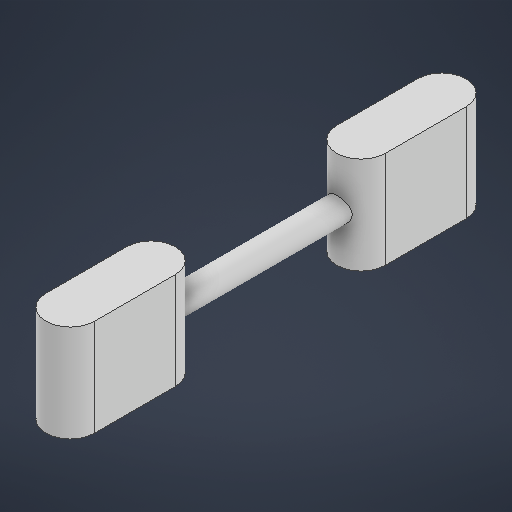
# Autodesk Inventor part: paletas
Saved by Autodesk Inventor 2025.3 (Build 293356000, 356)
## iProperties
Created: 2025-10-02
Part Number: paletas
Material: Generic
Document SubType Name: Modeling
Designer: sophi
Density: 1 g/cm^3
Appearance: Default
Author: sophi
Autodesk Inventor part; units mm, degrees
ref_plane "YZ Plane" through (0, 0, 0) normal (1, 0, 0) x (0, 1, 0)
ref_plane "XZ Plane" through (0, 0, 0) normal (0, 1, 0) x (-1, 0, 0)
ref_plane "XY Plane" through (0, 0, 0) normal (0, 0, 1) x (1, 0, 0)
sketch "Sketch1" plane through (0, 0, 0) normal (0, 1, 0) x (-1, 0, 0)
  line L0 (0, 23) -> (0, 13) construction
  line L1 (3, 23) -> (3, 13)
  line L2 (-3, 13) -> (-3, 23)
  arc A0 (3, 23) -> (-3, 23) centre (0, 23) ccw
  arc A1 (-3, 13) -> (3, 13) centre (0, 13) ccw
  line L3 (0, 30.2784) -> (0, -34.8413) construction
  line L4 (24.1166, 0) -> (-17.2731, 0) construction
  line L5 (0, 10) -> (0, -10)
  line L6 (3, -23) -> (3, -13)
  line L7 (-3, -13) -> (-3, -23)
  arc A2 (-3, -23) -> (3, -23) centre (0, -23) ccw
  arc A3 (3, -13) -> (-3, -13) centre (0, -13) ccw
  point P0 (0, 0)
  point P1 (0, 18)
  dimension "d0" = 10
  dimension "d1" = 3
  dimension "d2" = 20
  constraints: 18 end point, 9 point on circle, 7 symmetric about line, 5 point on line, 4 centre point, 4 tangent, 2 vertical, 1 horizontal, 1 midpoint, 1 parallel, 2 other
  measures "d0" distance of L0.start L0.end
  measures "d1" radius of A1
  measures "d2" distance of L5.start L5.end
extrude "Extrusion1" add sketch "Sketch1" along normal blind 12
ref_plane "Work Plane1" through (0, 12, -10) normal (0, 0, 1) x (1, 0, 0)
sketch "Sketch2" plane through (0, 12, -10) normal (0, 0, 1) x (1, 0, 0)
  circle A0 centre (0, -6) radius 1.5
  line L0 (3, 0) -> (-3, 0) projected
  line L1 (3, -12) -> (-3, -12) projected
  line L2 (3, -12) -> (3, 0) projected
  line L3 (-3, -12) -> (-3, 0) projected
  point P0 (0, -12)
  dimension "d5" = 3
  dimension "d6" = 6
  dimension "d7" = 3
  constraints: 1 centre point
  measures "d5" diameter of A0
  measures "d6" distance from line of A0.centre L0
  measures "d7" distance from line of L2 A0.centre
extrude "Extrusion2" add sketch "Sketch2" along normal blind 22 and the other way blind 2 contours A0
body "Solid1"
